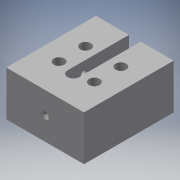
# Autodesk Inventor part: Mass 1
Saved by Autodesk Inventor 2016 (Build 200138000, 138)
## iProperties
Created: 2015-05-27
Part Number: Mass 1
Material: Steel, Mild
Document SubType Name: Modeling
Designer: Matthew Cheung
Density: 7.85 g/cm^3
Appearance: Steel
Mass: 367.007 g
Surface Area: 133.11 cm^2
Volume: 46.7525 cm^3
Author: Matthew Cheung
Autodesk Inventor part; units mm, degrees
ref_plane "YZ Plane" through (0, 0, 0) normal (1, 0, 0) x (0, 1, 0)
ref_plane "XZ Plane" through (0, 0, 0) normal (0, 1, 0) x (-1, 0, 0)
ref_plane "XY Plane" through (0, 0, 0) normal (0, 0, 1) x (1, 0, 0)
sketch "Sketch2" plane through (0, 0, 0) normal (0, 1, 0) x (-1, 0, 0)
  line L0 (-22, 25.4) -> (22, 25.4)
  line L1 (22, 25.4) -> (22, -25.4)
  line L2 (22, -25.4) -> (-22, -25.4)
  line L3 (-22, -25.4) -> (-22, 25.4)
  line L4 (-22, 25.4) -> (22, -25.4) construction
  line L5 (22, 25.4) -> (-22, -25.4) construction
  point P0 (0, 0)
  dimension "d0" = 50.8
  dimension "d1" = 44
  constraints: 12 end point, 2 midpoint, 2 parallel, 1 horizontal, 1 perpendicular
  measures "d0" distance of L0.end L1.end
  measures "d1" distance of L0.start L0.end
extrude "Extrusion1" add sketch "Sketch2" along normal blind 25.4
sketch "Sketch3" plane through (-22, 0, 25.4) normal (0, 0, 1) x (1, 0, 0)
  line L0 (0, 25.4) -> (44, 25.4) construction
  line L1 (0, 0) -> (44, 0) construction
  line L2 (44, 0) -> (44, 25.4) construction
  line L3 (44, 25.4) -> (0, 25.4) construction
  line L4 (0, 25.4) -> (0, 0) construction
  line L5 (0, 0) -> (44, 25.4) construction
  line L6 (44, 0) -> (0, 25.4) construction
  line L7 (44, 0) -> (0, 0) projected
  point P0 (22, 0)
  point P1 (22, 12.7)
  constraints: 12 end point, 2 midpoint, 2 parallel, 2 point on line, 1 horizontal, 1 perpendicular
hole "Hole1" at (0, 12.7, 25.4) direction (0, 0, -1) diameter 4.134 depth 12.7 tip angle 118 thread size "M5x0.8" class "6H" standard "ANSI Metric M Profile"
sketch "Sketch4" plane through (0, 25.4, 0) normal (0, 1, 0) x (1, 0, 0)
  line L0 (10, -7.5) -> (10, 7.5) construction
  line L1 (10, 7.5) -> (-10, 7.5) construction
  line L2 (-10, 7.5) -> (-10, -7.5) construction
  line L3 (-10, -7.5) -> (10, -7.5) construction
  line L4 (10, -7.5) -> (-10, 7.5) construction
  line L5 (10, 7.5) -> (-10, -7.5) construction
  circle A0 centre (-10, 7.5) radius 3
  circle A1 centre (10, 7.5) radius 3
  circle A2 centre (10, -7.5) radius 3
  circle A3 centre (-10, -7.5) radius 3
  point P0 (0, 0)
  dimension "d11" = 20
  dimension "d12" = 15
  dimension "d13" = 6
  dimension "d14" = 6
  dimension "d15" = 6
  dimension "d16" = 6
  constraints: 12 end point, 4 centre point, 4 coincident, 2 midpoint, 2 parallel, 1 perpendicular, 1 vertical
  measures "d11" distance of L0.end L1.end
  measures "d12" distance of L0.start L0.end
  measures "d13" diameter of A0
  measures "d14" diameter of A1
  measures "d15" diameter of A2
  measures "d16" diameter of A3
extrude "Extrusion2" cut sketch "Sketch4" against normal blind 5
sketch "Sketch5" plane through (-10, 20.4, 7.5) normal (0, 1, 0) x (1, 0, 0)
  circle A0 centre (0, 15) radius 3 projected
  circle A1 centre (20, 0) radius 3 projected
  circle A2 centre (20, 15) radius 3 projected
  point P0 (10, 7.5)
  point P1 (0, 0)
  constraints: 3 coincident
hole "Hole2" at (-10, 20.4, -7.5) at (-10, 20.4, 7.5) at (10, 20.4, 7.5) at (10, 20.4, -7.5) direction (0, -1, 0) diameter 3.5 end through all
sketch "Sketch8" plane through (-22, 0, -25.4) normal (-1, 0, 0) x (0, 0, 1)
  circle A0 centre (25.4, 19.05) radius 1.75
  line L0 (0, 25.4) -> (50.8, 25.4) projected
  line L1 (0, 0) -> (0, 25.4) projected
  circle A1 centre (25.4, 11.1125) radius 1.75
  arc A2 (28.4, 19.05) -> (22.4, 19.05) centre (25.4, 19.05) ccw
  arc A3 (22.4, 11.1125) -> (28.4, 11.1125) centre (25.4, 11.1125) ccw
  line L2 (28.4, 11.1125) -> (28.4, 19.05)
  line L3 (22.4, 19.05) -> (22.4, 11.1125)
  point P0 (25.4, 0)
  dimension "d31" = 3.5
  dimension "d32" = 6.35
  dimension "d33" = 25.4
  dimension "d41" = 3.5
  dimension "d42" = 7.9375
  dimension "d43" = 6
  dimension "d44" = 6
  constraints: 4 centre point, 4 end point, 4 point on circle, 2 coincident, 2 tangent, 1 vertical
  measures "d31" diameter of A0
  measures "d32" distance from line of L0 A0.centre
  measures "d33" distance from line of A0.centre L1
  measures "d41" diameter of A1
  measures "d42" distance of A1.centre A0.centre
  measures "d43" diameter of A2
  measures "d44" diameter of A3
extrude "Extrusion4" cut sketch "Sketch8" against normal blind 22 contours A0 | A1
sketch "Sketch9" plane through (22, 0, -25.4) normal (0, 0, -1) x (-1, 0, 0)
  line L0 (44, 25.4) -> (0, 25.4) projected
  line L1 (18.698, 25.4) -> (25.302, 25.4)
  line L2 (25.302, 25.4) -> (25.302, 6.35)
  line L3 (25.302, 6.35) -> (18.698, 6.35)
  line L4 (18.698, 6.35) -> (18.698, 25.4)
  line L5 (44, 0) -> (44, 25.4) projected
  point P0 (22, 0)
  point P1 (22, 6.35)
  dimension "d36" = 6.604
  dimension "d37" = 22
  dimension "d38" = 19.05
  constraints: 8 end point, 2 parallel, 1 horizontal, 1 midpoint, 1 perpendicular, 1 point on line
  measures "d36" distance of L2.end L3.end
  measures "d37" distance from line of L5 point (22, 6.35)
  measures "d38" distance of L1.end L2.end
extrude "Extrusion5" cut sketch "Sketch9" against normal blind 38.1
extrude "Extrusion6" cut sketch "Sketch8" against normal blind 3
fillet "Fillet1" radius 3.175 2 edges at (3.302, 15.875, 12.7) (-3.302, 15.875, 12.7)
body "Solid1"
